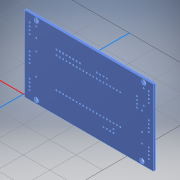
# Autodesk Inventor part: low_level_contoller_board.brd
Saved by Autodesk Inventor 2022 (Build 260153000, 153)
## iProperties
Created: 2022-12-23
Part Number: low_level_contoller_board.brd
Material: Типовые
Document SubType Name: Modeling
Designer: Ivan Petrov
Density: 1 g/cm^3
Appearance: Контур панели
Author: Ivan Petrov
Autodesk Inventor part; units mm, degrees
ref_plane "YZ Plane" through (0, 0, 0) normal (1, 0, 0) x (0, 1, 0)
ref_plane "XZ Plane" through (0, 0, 0) normal (0, 1, 0) x (-1, 0, 0)
ref_plane "XY Plane" through (0, 0, 0) normal (0, 0, 1) x (1, 0, 0)
sketch "Эскиз1" plane through (0, 0, 0) normal (0, 0, 1) x (1, 0, 0)
  line L0 (2.54, 15.24) -> (100, 15.24)
  line L1 (100, 15.24) -> (100, 72.38)
  line L2 (100, 72.38) -> (2.54, 72.38)
  line L3 (2.54, 72.38) -> (2.54, 15.24)
  circle A0 centre (6.35, 46.99) radius 0.51
  circle A1 centre (6.35, 44.45) radius 0.51
  circle A2 centre (6.35, 41.91) radius 0.51
  circle A3 centre (6.35, 39.37) radius 0.51
  circle A4 centre (96.52, 39.37) radius 0.51
  circle A5 centre (96.52, 41.91) radius 0.51
  circle A6 centre (96.52, 44.45) radius 0.51
  circle A7 centre (96.52, 46.99) radius 0.51
  circle A8 centre (6.35, 58.42) radius 0.51
  circle A9 centre (6.35, 60.96) radius 0.51
  circle A10 centre (6.35, 63.5) radius 0.51
  circle A11 centre (6.35, 66.04) radius 0.51
  circle A12 centre (6.35, 21.59) radius 0.51
  circle A13 centre (6.35, 24.13) radius 0.51
  circle A14 centre (6.35, 26.67) radius 0.51
  circle A15 centre (6.35, 29.21) radius 0.51
  circle A16 centre (96.52, 66.04) radius 0.51
  circle A17 centre (96.52, 63.5) radius 0.51
  circle A18 centre (96.52, 60.96) radius 0.51
  circle A19 centre (96.52, 58.42) radius 0.51
  circle A20 centre (96.52, 21.59) radius 0.51
  circle A21 centre (96.52, 24.13) radius 0.51
  circle A22 centre (96.52, 26.67) radius 0.51
  circle A23 centre (96.52, 29.21) radius 0.51
  circle A24 centre (69.85, 25.4) radius 0.51
  circle A25 centre (67.31, 25.4) radius 0.51
  circle A26 centre (64.77, 25.4) radius 0.51
  circle A27 centre (62.23, 25.4) radius 0.51
  circle A28 centre (87.63, 50.8) radius 0.51
  circle A29 centre (87.63, 53.34) radius 0.51
  circle A30 centre (87.63, 55.88) radius 0.51
  circle A31 centre (87.63, 58.42) radius 0.51
  circle A32 centre (57.15, 58.55) radius 0.51
  circle A33 centre (59.69, 58.55) radius 0.51
  circle A34 centre (62.23, 58.55) radius 0.51
  circle A35 centre (64.77, 58.55) radius 0.51
  circle A36 centre (26.67, 58.42) radius 0.6
  circle A37 centre (29.21, 58.42) radius 0.6
  circle A38 centre (31.75, 58.42) radius 0.6
  circle A39 centre (34.29, 58.42) radius 0.6
  circle A40 centre (36.83, 58.42) radius 0.6
  circle A41 centre (39.37, 58.42) radius 0.6
  circle A42 centre (41.91, 58.42) radius 0.6
  circle A43 centre (44.45, 58.42) radius 0.6
  circle A44 centre (36.83, 31.75) radius 0.5
  circle A45 centre (39.37, 31.75) radius 0.5
  circle A46 centre (41.91, 31.75) radius 0.5
  circle A47 centre (44.45, 31.75) radius 0.5
  circle A48 centre (31.75, 31.75) radius 0.5
  circle A49 centre (46.99, 31.75) radius 0.5
  circle A50 centre (49.53, 31.75) radius 0.5
  circle A51 centre (29.21, 31.75) radius 0.5
  circle A52 centre (72.39, 54.61) radius 0.5
  circle A53 centre (52.07, 31.75) radius 0.5
  circle A54 centre (54.61, 31.75) radius 0.5
  circle A55 centre (57.15, 31.75) radius 0.5
  circle A56 centre (59.69, 31.75) radius 0.5
  circle A57 centre (62.23, 31.75) radius 0.5
  circle A58 centre (64.77, 31.75) radius 0.5
  circle A59 centre (67.31, 31.75) radius 0.5
  circle A60 centre (69.85, 31.75) radius 0.5
  circle A61 centre (72.39, 31.75) radius 0.5
  circle A62 centre (74.93, 31.75) radius 0.5
  circle A63 centre (46.99, 54.61) radius 0.5
  circle A64 centre (49.53, 54.61) radius 0.5
  circle A65 centre (52.07, 54.61) radius 0.5
  circle A66 centre (54.61, 54.61) radius 0.5
  circle A67 centre (57.15, 54.61) radius 0.5
  circle A68 centre (59.69, 54.61) radius 0.5
  circle A69 centre (62.23, 54.61) radius 0.5
  circle A70 centre (64.77, 54.61) radius 0.5
  circle A71 centre (67.31, 54.61) radius 0.5
  circle A72 centre (69.85, 54.61) radius 0.5
  circle A73 centre (74.93, 54.61) radius 0.5
  circle A74 centre (39.37, 54.61) radius 0.5
  circle A75 centre (34.29, 31.75) radius 0.5
  circle A76 centre (31.75, 54.61) radius 0.5
  circle A77 centre (34.29, 54.61) radius 0.5
  circle A78 centre (44.45, 54.61) radius 0.5
  circle A79 centre (26.67, 31.75) radius 0.5
  circle A80 centre (36.83, 54.61) radius 0.5
  circle A81 centre (26.67, 54.61) radius 0.5
  circle A82 centre (29.21, 54.61) radius 0.5
  circle A83 centre (41.91, 54.61) radius 0.5
  circle A84 centre (11.43, 17.78) radius 1.75
  circle A85 centre (91.44, 17.78) radius 1.75
  circle A86 centre (92.71, 69.85) radius 1.75
  circle A87 centre (11.43, 69.85) radius 1.75
  circle A88 centre (11.43, 66.04) radius 0.5
  circle A89 centre (11.43, 58.42) radius 0.5
  circle A90 centre (11.43, 49.53) radius 0.5
  circle A91 centre (11.43, 33.02) radius 0.5
  circle A92 centre (92.71, 66.04) radius 0.5
  circle A93 centre (92.71, 54.61) radius 0.5
  circle A94 centre (91.44, 50.8) radius 0.5
  circle A95 centre (91.44, 36.83) radius 0.5
  circle A96 centre (91.44, 29.21) radius 0.5
  circle A97 centre (69.85, 27.94) radius 0.5
  constraints: 98 centre point, 8 end point
extrude "low_level_contoller_board.brdКонтур" add sketch "Эскиз1" along normal blind 1.6
